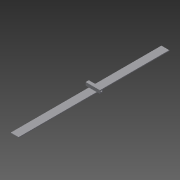
# Autodesk Inventor part: Part2
Saved by Autodesk Inventor 2014 SP1 (Build 180222100, 222)
## iProperties
Created: 2018-05-14
Part Number: Part2
Material: Generic
Document SubType Name: Modeling
Designer: Dadang
Density: 1 g/cm^3
Appearance: Default
Author: Dadang
Autodesk Inventor part; units mm, degrees
ref_plane "YZ Plane" through (0, 0, 0) normal (1, 0, 0) x (0, 1, 0)
ref_plane "XZ Plane" through (0, 0, 0) normal (0, 1, 0) x (-1, 0, 0)
sketch "Sketch1" plane through (0, 0, 0) normal (0, 0, 1) x (1, 0, 0)
  line L0 (0, 0) -> (50, 0)
  line L1 (50, 0) -> (50, 5)
  line L2 (50, 5) -> (0, 5)
  line L3 (0, 5) -> (0, 0)
  dimension "d0" = 50
  dimension "d1" = 5
  constraints: 8 end point, 2 parallel, 1 horizontal, 1 perpendicular
  measures "d0" distance of L2.end L1.end
  measures "d1" distance of L1.end L0.end
extrude "Extrusion1" add sketch "Sketch1" along normal blind 955
ref_plane "Work Plane1" through (0, 0, 0) normal (0, 0, 1) x (1, 0, 0)
sketch "Sketch3" plane through (0, 0, 0) normal (0, 0, 1) x (1, 0, 0)
  line L0 (0, 0) -> (50, 0) projected
  line L1 (0, 5) -> (0, 0) projected
  line L2 (50, 5) -> (0, 5) projected
  line L3 (50, 0) -> (50, 5) projected
  line L4 (0, 5) -> (50, 5) projected
  line L5 (0, 5) -> (0, 25) projected
  line L6 (50, 25) -> (0, 25) projected
  line L7 (50, 5) -> (50, 25) projected
sketch "Sketch5" plane through (0, 5, 0) normal (0, 1, 0) x (1, 0, 0)
  line L0 (70, -440) -> (70, -460)
  line L1 (-20, -440) -> (-20, -460)
  line L2 (50, 0) -> (0, 0) projected
  line L3 (-20, -460) -> (70, -460)
  line L4 (-20, -440) -> (70, -440)
  point P0 (50, -450)
  dimension "d33" = 20
  constraints: 8 end point, 2 parallel
  measures "d33" distance of L0.start L0.end
extrude "Extrusion7" add sketch "Sketch5" along normal blind 20
sketch "Sketch7" plane through (70, 5, 460) normal (1, 0, 0) x (0, 0, -1)
  circle A0 centre (10, 10) radius 5
  point P0 (460, -5)
  dimension "d39" = 10
  constraints: 1 centre point
  measures "d39" diameter of A0
extrude "Extrusion8" cut sketch "Sketch7" against normal blind 100
body "Solid1"
